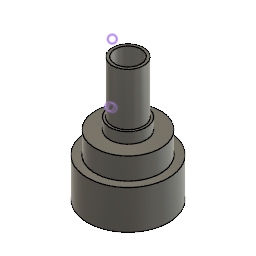
Bike Pump 3D v1 (Autodesk Fusion 360 design; units mm, degrees)
Autodesk Fusion 360 part; units mm, degrees
sketch "Sketch1" plane through (0, 0, 0) normal (0, 1, 0) x (1, 0, 0)
  circle A0 centre (0, 0) radius 10.375
  circle A1 centre (0, 0) radius 11.175
  circle A2 centre (0, 0) radius 7.625
  circle A3 centre (0, 0) radius 6.825
  dimension "d1" = 20.75
  dimension "d2" = 22.35
  dimension "d3" = 15.25
  dimension "d4" = 13.65
  constraint coincident A0.centre A1.centre
  constraint concentric A1 A2
  constraint concentric A2 A3
  measures "d1" diameter of A0
  measures "d2" diameter of A1
  measures "d3" diameter of A2
  measures "d4" diameter of A3
extrude "Extrude1" add sketch "Sketch1" along normal blind 5.75 makes body 1 at (7.6155, 3.8333, 0.3801) makes body 2 at (11.1611, 3.8333, 0.557)
extrude "Extrude2" cut 1 faces at (7.3045, 0, 0.7179) along direction (0, 1, 0) blind 1 on bodies 1 bodies 1
sketch "Sketch2" plane through (0, 5.75, 0) normal (0, 1, 0) x (-1, 0, 0)
  circle A0 centre (0, 0) radius 10.375
  circle A1 centre (0, 0) radius 11.175
  circle A2 centre (0, 0) radius 11.175
  circle A3 centre (0, 0) radius 6.825
  circle A4 centre (0, 0) radius 6.825
  constraint coincident A0.centre A1.centre
extrude "Extrude3" add sketch "Sketch2" along normal blind 5 contours A0 | A1 A2 bodies 1 2
sketch "Sketch3" plane through (0, 0, 0) normal (0, 1, 0) x (1, 0, 0)
sketch "Sketch4" plane through (0, 0, 0) normal (0, 1, 0) x (1, 0, 0)
  circle A0 centre (0, 0) radius 9
  circle A1 centre (0, 0) radius 4.375
  dimension "d11" = 8.75
  constraint coincident A0.centre A1.centre
  measures "d11" diameter of A1
extrude "Extrude4" add sketch "Sketch4" along normal blind 6 from surface at 10.75 bodies 1
fillet "Fillet1" radius 4.9 1 edges at (-4.0789, 10.75, 1.5821) on bodies 1
sketch "Sketch5" plane through (0, 0, 0) normal (0, 1, 0) x (1, 0, 0)
  circle A0 centre (0, 0) radius 3.575
  circle A1 centre (0, 0) radius 5
  dimension "d17" = 7.15
  constraint coincident A0.centre A1.centre
  measures "d17" diameter of A0
extrude "Extrude5" add sketch "Sketch5" along normal blind 3 from surface at 16.75 bodies 1
sketch "Sketch6" plane through (0, 0, 0) normal (0, 1, 0) x (1, 0, 0)
  circle A0 centre (0, 0) radius 4.35
  circle A1 centre (0, 0) radius 3.575
  dimension "d21" = 8.7
  dimension "d22" = 7.15
  constraint coincident A0.centre A1.centre
  measures "d21" diameter of A0
  measures "d22" diameter of A1
extrude "Extrude6" add sketch "Sketch6" along normal blind 16.45 from surface at 19.75 bodies 1
sketch "Sketch7" plane through (0, 0, 0) normal (0, 0, 1) x (1, 0, 0)
sketch "Sketch8" plane through (0, 0, 0) normal (0, 0, 1) x (1, 0, 0)
sketch "Sketch9" plane through (0, 0, 0) normal (0, 0, 1) x (1, 0, 0)
  point P0 (-4.35, 36.2)
  point P1 (-5, 19.75)
  point P2 (-4.35, 19.75)
extrude "Extrude7" cut 1 faces at (4.0755, 36.2, 0.2161) along direction (0, -1, 0) blind 2 on bodies 1 bodies 1
extrude "Extrude8" add 1 faces at (7.3045, 1, 0.7179) along direction (0, -1, 0) blind 1 on bodies 1 bodies 1
